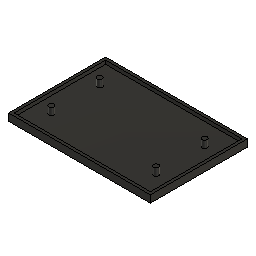
mounting_base_xl4016 (Autodesk Fusion 360 design; units mm, degrees)
Autodesk Fusion 360 part; units mm, degrees
sketch "Sketch1" plane through (0, 0, 0) normal (0, 0, 1) x (1, 0, 0)
  line L0 (0, 0) -> (65.5, 0)
  line L1 (65.5, 0) -> (65.5, 36.7)
  line L2 (65.5, 36.7) -> (0, 36.7)
  line L3 (0, 36.7) -> (0, 0)
  line L4 (0, 0) -> (0, 2)
  line L5 (-5, -5) -> (70.5, -5)
  line L6 (70.5, -5) -> (70.5, 41.7)
  line L7 (70.5, 41.7) -> (-5, 41.7)
  line L8 (-5, 41.7) -> (-5, -5)
  line L9 (72, 43.2) -> (-6.5, 43.2)
  line L10 (-6.5, 43.2) -> (-6.5, -6.5)
  line L11 (-6.5, -6.5) -> (72, -6.5)
  line L12 (72, -6.5) -> (72, 43.2)
  line L13 (0, 0) -> (0, 5)
  line L14 (0, 36.7) -> (3.7, 36.7)
  line L15 (3.7, 36.7) -> (3.7, 31.7)
  line L16 (3.7, 31.7) -> (0, 31.7)
  line L17 (0, 31.7) -> (0, 36.7)
  line L18 (65.5, 36.7) -> (61.8, 36.7)
  line L19 (61.8, 36.7) -> (61.8, 31.7)
  line L20 (61.8, 31.7) -> (65.5, 31.7)
  line L21 (65.5, 31.7) -> (65.5, 36.7)
  line L22 (65.5, 0) -> (61.8, 0)
  line L23 (61.8, 0) -> (61.8, 5)
  line L24 (61.8, 5) -> (65.5, 5)
  line L25 (65.5, 5) -> (65.5, 0)
  circle A0 centre (3.7, 31.7) radius 1.4
  circle A1 centre (61.8, 31.7) radius 1.4
  circle A2 centre (61.8, 5) radius 1.4
  line L26 (0, 5) -> (3.7, 5)
  circle A3 centre (3.7, 5) radius 1.4
  dimension "d1" = 65.5
  dimension "d2" = 36.7
  dimension "d8" = 5
  dimension "d9" = 1.5
  dimension "d18" = 5
  dimension "d21" = 3.7
  dimension "d22" = 5
  dimension "d23" = 3.7
  dimension "d24" = 5
  dimension "d25" = 3.7
  dimension "d26" = 5
  dimension "d27" = 2.8
  dimension "d28" = 2.8
  dimension "d29" = 2.8
  dimension "d39" = 3.7
  dimension "d40" = 2.8
  constraint horizontal L0
  constraint vertical L1
  constraint horizontal L2
  constraint vertical L3
  constraint coincident L0.start L3.end
  constraint coincident L3 L4.end
  constraint perpendicular L0 L13
  constraint horizontal L14
  constraint vertical L15
  constraint horizontal L16
  constraint vertical L17
  constraint horizontal L18
  constraint vertical L19
  constraint horizontal L20
  constraint vertical L21
  constraint horizontal L22
  constraint vertical L23
  constraint horizontal L24
  constraint vertical L25
  constraint coincident L15.end L16.start
  constraint coincident L19.end L20.start
  constraint coincident L23.end L24.start
  constraint coincident L26.end A3.centre
  measures "d1" distance of L0.start L0.end
  measures "d2" distance of L0.start L2.end
  measures "d18" distance of L0.start L13.end
  measures "d21" distance of L2.end L14.end
  measures "d22" distance of L2.end L16.end
  measures "d23" distance of L1.end L18.end
  measures "d24" distance of L1.end L20.end
  measures "d25" distance of L0.end L22.end
  measures "d26" distance of L0.end L24.end
  measures "d27" diameter of A0
  measures "d28" diameter of A1
  measures "d29" diameter of A2
  measures "d39" distance of L13.end L26.end
  measures "d40" diameter of A3
extrude "Extrude1" add sketch "Sketch1" against normal blind 2 contours L0 L1 L2 L3 L4 L13 L15 L16 L19 L20 L23 L24 A0 A1 A2 | L0 L1 L22 L23 L24 L25 A2 | L23 L24 A2 | L23 L24 A2 | L2 L3 L14 L15 L16 L17 A0 | L1 L2 L18 L19 L20 L21 A1 | L15 L16 A0 | L15 L16 A0 | L19 L20 A1 | L19 L20 A1 | L5 L6 L7 L8 | L9 L10 L11 L12 | A3
extrude "Extrude3" add sketch "Sketch1" along normal blind 2 contours L9 L10 L11 L12
extrude "Extrude4" add sketch "Sketch1" along normal blind 4 contours L23 L24 A2 | L23 L24 A2 | L15 L16 A0 | L15 L16 A0 | L19 L20 A1 | L19 L20 A1
move_face "OffsetFaces1" offset 2 2 faces at (45.8333, 43.2, -0.6667) (45.8333, -6.5, -0.6667)
move_face "OffsetFaces2" offset -2 2 faces at (20.1667, -5, 0.6667) (45.3333, 41.7, 0.6667)
extrude "Extrude6" add sketch "Sketch1" along normal blind 4 contours A3
